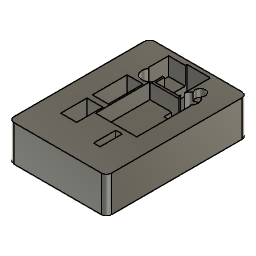
soldering jig v4 (Autodesk Fusion 360 design; units mm, degrees)
Autodesk Fusion 360 part; units mm, degrees
(part 1 of 4)
sketch "Universal_Board_Side_Mount" plane through (0, 0, 0) normal (0, 0, 1) x (1, 0, 0)
  arc A0 (2.8448, 30.9521) -> (2.7093, 31.3585) centre (2.1675, 30.9521) ccw
  arc A1 (2.2648, 29.4642) -> (2.341, 29.4642) centre (2.3029, 29.4642) ccw
  arc A2 (2.1675, 30.7715) -> (2.4836, 30.5909) centre (2.4836, 30.9577) ccw
  arc A3 (1.2192, 29.9158) -> (1.4901, 29.6448) centre (1.4902, 29.9158) ccw
  arc A4 (1.2573, 29.9158) -> (1.1811, 29.9158) centre (1.2192, 29.9158) ccw
  arc A5 (1.5804, 31.4107) -> (1.5804, 31.4869) centre (1.5804, 31.4488) ccw
  arc A6 (1.5804, 31.4488) -> (1.2192, 31.0876) centre (1.5804, 31.0876) ccw
  arc A7 (1.8637, 31.2489) -> (1.9294, 31.2875) centre (1.8965, 31.2682) ccw
  arc A8 (2.4836, 23.7652) -> (2.8448, 24.1265) centre (2.4835, 24.1265) ccw
  line L0 (2.8448, 29.6448) -> (1.4901, 29.6448)
  arc A9 (2.4836, 30.5909) -> (2.8448, 30.9521) centre (2.4836, 30.9521) ccw
  arc A10 (2.4836, 30.5528) -> (2.4836, 30.629) centre (2.4836, 30.5909) ccw
  arc A11 (2.4836, 23.8033) -> (2.4836, 23.7271) centre (2.4836, 23.7652) ccw
  arc A12 (1.2192, 31.0876) -> (1.445, 30.5457) centre (1.9824, 31.0876) ccw
  arc A13 (2.8067, 24.1265) -> (2.8829, 24.1265) centre (2.8448, 24.1265) ccw
  arc A14 (1.8965, 31.2682) -> (1.5804, 31.4488) centre (1.5804, 31.082) ccw
  arc A15 (1.4901, 29.6829) -> (1.4901, 29.6067) centre (1.4901, 29.6448) ccw
  arc A16 (2.8448, 29.6067) -> (2.8448, 29.6829) centre (2.8448, 29.6448) ccw
  arc A17 (1.4901, 29.6067) -> (1.4901, 29.6829) centre (1.4901, 29.6448) ccw
  arc A18 (1.4901, 32.7867) -> (1.4901, 32.8629) centre (1.4901, 32.8248) ccw
  line L1 (1.2192, 29.9158) -> (1.2192, 30.0061)
  arc A19 (1.2573, 30.0061) -> (1.1811, 30.0061) centre (1.2192, 30.0061) ccw
  arc A20 (1.1811, 31.0876) -> (1.2573, 31.0876) centre (1.2192, 31.0876) ccw
  arc A21 (2.8829, 24.1265) -> (2.8067, 24.1265) centre (2.8448, 24.1265) ccw
  arc A22 (2.8448, 24.1265) -> (2.7093, 24.5329) centre (2.1675, 24.1265) ccw
  arc A23 (2.7398, 24.5557) -> (2.6789, 24.51) centre (2.7093, 24.5329) ccw
  arc A24 (1.1811, 29.9158) -> (1.2573, 29.9158) centre (1.2192, 29.9158) ccw
  arc A25 (1.1811, 24.262) -> (1.2573, 24.262) centre (1.2192, 24.262) ccw
  arc A26 (2.4836, 23.7271) -> (2.4836, 23.8033) centre (2.4836, 23.7652) ccw
  arc A27 (2.4836, 30.629) -> (2.4836, 30.5528) centre (2.4836, 30.5909) ccw
  arc A28 (2.2003, 23.9652) -> (2.1346, 23.9265) centre (2.1675, 23.9459) ccw
  arc A29 (1.2192, 24.262) -> (1.445, 23.7201) centre (1.9824, 24.262) ccw
  arc A30 (2.8067, 30.9521) -> (2.8829, 30.9521) centre (2.8448, 30.9521) ccw
  arc A31 (1.4181, 23.693) -> (1.4718, 23.7471) centre (1.445, 23.7201) ccw
  arc A32 (2.032, 34.8114) -> (2.032, 34.8876) centre (2.032, 34.8495) ccw
  line L2 (2.8448, 33.4913) -> (2.7545, 33.4913)
  arc A33 (2.341, 32.5538) -> (2.2648, 32.5538) centre (2.3029, 32.5538) ccw
  arc A34 (2.3029, 34.5786) -> (2.032, 34.8495) centre (2.032, 34.5786) ccw
  arc A35 (2.8448, 33.4532) -> (2.8448, 33.5294) centre (2.8448, 33.4913) ccw
  arc A36 (1.969, 37.4483) -> (2.0047, 37.5157) centre (1.9868, 37.482) ccw
  arc A37 (1.5804, 24.6613) -> (1.5804, 24.5851) centre (1.5804, 24.6232) ccw
  arc A38 (2.134, 23.9276) -> (2.2009, 23.9641) centre (2.1674, 23.9459) ccw
  arc A39 (2.8067, 36.0444) -> (2.8829, 36.0444) centre (2.8448, 36.0444) ccw
  line L3 (2.3029, 34.127) -> (2.3029, 34.5786)
  arc A40 (2.1675, 23.9459) -> (2.4836, 23.7652) centre (2.4836, 24.1321) ccw
  arc A41 (1.2072, 39.6306) -> (1.2312, 39.5583) centre (1.2192, 39.5945) ccw
  arc A42 (2.4384, 36.4508) -> (2.1223, 36.3154) centre (2.4383, 36.0144) ccw
  line L4 (2.3029, 37.8884) -> (1.7611, 37.1659)
  arc A43 (2.341, 34.5786) -> (2.2648, 34.5786) centre (2.3029, 34.5786) ccw
  arc A44 (2.4718, 35.5839) -> (2.4953, 35.5115) centre (2.4836, 35.5477) ccw
  arc A45 (2.8829, 36.0444) -> (2.8067, 36.0444) centre (2.8448, 36.0444) ccw
  arc A46 (1.5804, 24.5851) -> (1.5804, 24.6613) centre (1.5804, 24.6232) ccw
  arc A47 (2.3029, 34.0889) -> (2.3029, 34.1651) centre (2.3029, 34.127) ccw
  arc A48 (2.8448, 41.0464) -> (2.4384, 41.4528) centre (2.4384, 41.0464) ccw
  line L5 (2.1223, 36.3154) -> (1.2192, 35.5477)
  arc A49 (1.1945, 35.5767) -> (1.2439, 35.5187) centre (1.2192, 35.5477) ccw
  arc A50 (2.4384, 36.4127) -> (2.4384, 36.4889) centre (2.4384, 36.4508) ccw
  arc A51 (2.0947, 36.3416) -> (2.1499, 36.2891) centre (2.1223, 36.3154) ccw
  arc A52 (2.7164, 33.401) -> (2.7926, 33.401) centre (2.7545, 33.401) ccw
  arc A53 (1.8637, 24.4232) -> (1.9294, 24.4619) centre (1.8966, 24.4426) ccw
  arc A54 (2.8067, 41.0464) -> (2.8829, 41.0464) centre (2.8448, 41.0464) ccw
  arc A55 (2.032, 34.8876) -> (2.032, 34.8114) centre (2.032, 34.8495) ccw
  line L6 (1.2192, 37.1659) -> (2.8448, 37.1659)
  arc A56 (2.3334, 37.8655) -> (2.2725, 37.9113) centre (2.303, 37.8884) ccw
  line L7 (2.8448, 33.401) -> (2.8448, 33.4913)
  arc A57 (2.7545, 33.4391) -> (2.7545, 33.3629) centre (2.7545, 33.401) ccw
  line L8 (2.032, 34.8495) -> (1.2192, 34.8495)
  arc A58 (2.2648, 34.127) -> (2.341, 34.127) centre (2.3029, 34.127) ccw
  arc A59 (2.4718, 40.5859) -> (2.4953, 40.5134) centre (2.4836, 40.5496) ccw
  arc A60 (1.5804, 24.6232) -> (1.2192, 24.262) centre (1.5804, 24.262) ccw
  line L9 (1.2192, 39.5944) -> (2.3029, 39.9557)
  line L10 (1.8965, 24.4426) -> (2.1675, 23.9459)
  arc A61 (2.8067, 33.401) -> (2.8829, 33.401) centre (2.8448, 33.401) ccw
  arc A62 (1.8965, 24.4426) -> (1.5804, 24.6232) centre (1.5804, 24.2564) ccw
  arc A63 (1.4901, 32.8629) -> (1.4901, 32.7867) centre (1.4901, 32.8248) ccw
  arc A64 (2.8448, 33.3629) -> (2.8448, 33.4391) centre (2.8448, 33.401) ccw
  arc A65 (2.7545, 33.5294) -> (2.7545, 33.4532) centre (2.7545, 33.4913) ccw
  arc A66 (1.93, 31.2865) -> (1.8631, 31.25) centre (1.8966, 31.2682) ccw
  arc A67 (1.2312, 39.6306) -> (1.2072, 39.5583) centre (1.2192, 39.5945) ccw
  arc A68 (1.2573, 24.262) -> (1.1811, 24.2619) centre (1.2192, 24.2619) ccw
  arc A69 (2.4384, 41.4909) -> (2.4384, 41.4147) centre (2.4384, 41.4528) ccw
  line L11 (2.3029, 39.2332) -> (1.2192, 39.5944)
  arc A70 (2.4836, 35.5477) -> (2.8448, 36.0444) centre (2.3227, 36.0444) ccw
  arc A71 (2.4836, 40.5497) -> (2.8448, 41.0464) centre (2.3227, 41.0464) ccw
  arc A72 (2.4384, 36.4889) -> (2.4384, 36.4127) centre (2.4384, 36.4508) ccw
  arc A73 (1.2192, 37.204) -> (1.2192, 37.1278) centre (1.2192, 37.1659) ccw
  arc A74 (11.3867, 7.6438) -> (11.3674, 7.6766) centre (11.3771, 7.6602) ccw
  arc A75 (1.237, 37.9221) -> (1.2014, 37.8547) centre (1.2192, 37.8884) ccw
  line L12 (11.3771, 7.6602) -> (11.6021, 7.783)
  arc A76 (2.4384, 41.4147) -> (2.4384, 41.4909) centre (2.4384, 41.4528) ccw
  arc A77 (1.7306, 37.1888) -> (1.7915, 37.1431) centre (1.761, 37.1659) ccw
  arc A78 (11.3143, 7.517) -> (11.2762, 7.517) centre (11.2953, 7.517) ccw
  arc A79 (1.2192, 34.8876) -> (1.2192, 34.8114) centre (1.2192, 34.8495) ccw
  line L13 (1.2192, 35.5477) -> (1.2192, 36.4508)
  line L14 (29.1592, 41.6532) -> (28.3803, 41.6532)
  arc A80 (11.3247, 8.0438) -> (11.3476, 8.0133) centre (11.3361, 8.0285) ccw
  arc A81 (11.3771, 7.6602) -> (11.2952, 7.517) centre (11.4614, 7.5169) ccw
  arc A82 (24.7438, 43.7776) -> (24.7438, 43.7395) centre (24.7438, 43.7585) ccw
  line L15 (25.2349, 43.7586) -> (24.7438, 43.7586)
  arc A83 (2.7926, 33.4913) -> (2.7164, 33.4913) centre (2.7545, 33.4913) ccw
  arc A84 (11.718, 7.4422) -> (11.6909, 7.469) centre (11.7044, 7.4556) ccw
  line L16 (24.9894, 43.513) -> (24.9894, 44.0041)
  line L17 (11.9084, 40.084) -> (11.9084, 40.5751)
  arc A85 (2.0947, 41.3436) -> (2.1499, 41.2911) centre (2.1223, 41.3173) ccw
  line L18 (2.1223, 41.3173) -> (1.2192, 40.5497)
  line L19 (1.2192, 40.5497) -> (1.2192, 41.4528)
  arc A86 (2.315, 39.9195) -> (2.2909, 39.9918) centre (2.303, 39.9557) ccw
  arc A87 (1.1811, 40.5497) -> (1.2573, 40.5497) centre (1.2192, 40.5497) ccw
  arc A88 (28.3803, 43.8376) -> (28.3803, 43.7868) centre (28.3803, 43.8122) ccw
  arc A89 (2.3029, 33.4081) -> (2.3029, 33.4843) centre (2.3029, 33.4462) ccw
  arc A90 (2.8448, 36.0444) -> (2.4384, 36.4508) centre (2.4384, 36.0444) ccw
  arc A91 (24.8539, 41.9615) -> (24.8539, 41.9996) centre (24.8539, 41.9806) ccw
  arc A92 (11.8893, 40.084) -> (11.9274, 40.084) centre (11.9084, 40.084) ccw
  arc A93 (25.0084, 44.0041) -> (24.9703, 44.0041) centre (24.9894, 44.0041) ccw
  line L20 (29.1592, 43.8122) -> (28.3803, 43.8122)
  arc A94 (28.3803, 41.6786) -> (28.3803, 41.6278) centre (28.3803, 41.6532) ccw
  arc A95 (2.2648, 34.5786) -> (2.341, 34.5786) centre (2.3029, 34.5786) ccw
  arc A96 (2.8829, 33.4913) -> (2.8067, 33.4913) centre (2.8448, 33.4913) ccw
  arc A97 (29.1592, 41.6278) -> (29.1592, 41.6786) centre (29.1592, 41.6532) ccw
  arc A98 (24.9703, 43.513) -> (25.0084, 43.513) centre (24.9894, 43.513) ccw
  arc A99 (1.2573, 36.4508) -> (1.1811, 36.4508) centre (1.2192, 36.4508) ccw
  arc A100 (11.5925, 7.7994) -> (11.6118, 7.7666) centre (11.6021, 7.783) ccw
  arc A101 (12.1539, 40.3105) -> (12.1539, 40.3486) centre (12.1539, 40.3295) ccw
  arc A102 (9.2329, 45.7715) -> (9.2329, 45.8096) centre (9.2329, 45.7906) ccw
  line L21 (1.2192, 37.8884) -> (1.9868, 37.482)
  arc A103 (1.1811, 35.5477) -> (1.2573, 35.5477) centre (1.2192, 35.5477) ccw
  arc A104 (11.6113, 7.7663) -> (11.593, 7.7997) centre (11.6021, 7.783) ccw
  arc A105 (24.6274, 42.2261) -> (24.5893, 42.2261) centre (24.6084, 42.2261) ccw
  arc A106 (11.6628, 40.3486) -> (11.6628, 40.3105) centre (11.6628, 40.3295) ccw
  arc A107 (1.2573, 41.4528) -> (1.1811, 41.4528) centre (1.2192, 41.4528) ccw
  arc A108 (2.8448, 37.1278) -> (2.8448, 37.204) centre (2.8448, 37.1659) ccw
  line L22 (1.2192, 34.127) -> (2.3029, 34.127)
  arc A109 (29.1592, 43.7868) -> (29.1592, 43.8376) centre (29.1592, 43.8122) ccw
  arc A110 (2.8829, 41.0464) -> (2.8067, 41.0464) centre (2.8448, 41.0464) ccw
  line L23 (2.7545, 33.401) -> (2.8448, 33.401)
  arc A111 (25.2349, 43.7395) -> (25.2349, 43.7776) centre (25.2349, 43.7585) ccw
  line L24 (2.7545, 33.4913) -> (2.7545, 33.401)
  arc A112 (24.3628, 41.9996) -> (24.3628, 41.9615) centre (24.3628, 41.9806) ccw
  line L25 (7.9629, 42.3616) -> (7.4718, 42.3616)
  arc A113 (7.4718, 42.3806) -> (7.4718, 42.3425) centre (7.4718, 42.3616) ccw
  arc A114 (2.2909, 39.197) -> (2.315, 39.2693) centre (2.303, 39.2332) ccw
  arc A115 (11.3679, 7.6769) -> (11.3862, 7.6435) centre (11.3771, 7.6602) ccw
  arc A116 (1.2192, 34.1651) -> (1.2192, 34.0889) centre (1.2192, 34.127) ccw
  arc A117 (2.147, 36.2863) -> (2.0976, 36.3444) centre (2.1223, 36.3154) ccw
  arc A118 (11.2762, 7.517) -> (11.3143, 7.517) centre (11.2953, 7.517) ccw
  line L26 (24.6084, 41.735) -> (24.6084, 42.2261)
  arc A119 (1.2192, 33.4843) -> (1.2192, 33.4081) centre (1.2192, 33.4462) ccw
  line L27 (9.2329, 45.7906) -> (8.7418, 45.7906)
  line L28 (9.8677, 8.0899) -> (9.8268, 8.0899)
  arc A120 (10.3484, 7.8444) -> (10.3103, 7.8444) centre (10.3294, 7.8444) ccw
  arc A121 (7.9629, 42.3425) -> (7.9629, 42.3806) centre (7.9629, 42.3616) ccw
  arc A122 (11.6649, 7.9262) -> (11.703, 7.9262) centre (11.6839, 7.9262) ccw
  arc A123 (8.8056, 7.6807) -> (8.8437, 7.6807) centre (8.8247, 7.6807) ccw
  line L29 (7.9629, 15.9456) -> (7.4718, 15.9456)
  arc A124 (11.5203, 8.0709) -> (11.5203, 8.1089) centre (11.5203, 8.0899) ccw
  arc A125 (11.4589, 7.3723) -> (11.4589, 7.3343) centre (11.4589, 7.3533) ccw
  arc A126 (9.4328, 7.3723) -> (9.4328, 7.3342) centre (9.4328, 7.3533) ccw
  arc A127 (9.5774, 7.4761) -> (9.6155, 7.4761) centre (9.5965, 7.4761) ccw
  arc A128 (9.152, 7.6807) -> (8.8246, 7.6807) centre (8.9883, 7.6807) ccw
  arc A129 (11.6021, 7.783) -> (11.684, 7.9262) centre (11.5178, 7.9263) ccw
  arc A130 (1.1945, 40.5787) -> (1.2439, 40.5207) centre (1.2192, 40.5497) ccw
  arc A131 (10.7761, 7.8253) -> (10.7762, 7.8634) centre (10.7761, 7.8444) ccw
  line L30 (8.8246, 7.6807) -> (8.8246, 7.5988)
  arc A132 (11.684, 7.9262) -> (11.5203, 8.0899) centre (11.5203, 7.9262) ccw
  arc A133 (11.2952, 7.517) -> (11.4589, 7.3533) centre (11.4589, 7.517) ccw
  line L31 (24.8539, 41.9806) -> (24.3628, 41.9806)
  line L32 (10.3294, 7.3533) -> (10.3294, 7.8444)
  arc A134 (9.171, 7.6807) -> (9.1329, 7.6807) centre (9.1519, 7.6807) ccw
  line L33 (12.1539, 40.3296) -> (11.6628, 40.3296)
  arc A135 (10.3103, 7.3533) -> (10.3484, 7.3533) centre (10.3294, 7.3533) ccw
  arc A136 (9.9714, 7.3533) -> (10.0095, 7.3533) centre (9.9904, 7.3533) ccw
  arc A137 (10.6724, 7.7216) -> (10.6343, 7.7216) centre (10.6534, 7.7216) ccw
  line L34 (9.9904, 7.3533) -> (9.9904, 7.9671)
  line L35 (10.6534, 7.7216) -> (10.6534, 7.3533)
  arc A138 (8.7418, 45.8096) -> (8.7418, 45.7715) centre (8.7418, 45.7906) ccw
  arc A139 (7.4718, 15.9646) -> (7.4718, 15.9265) centre (7.4718, 15.9455) ccw
  arc A140 (9.4328, 7.8634) -> (9.4328, 7.8253) centre (9.4328, 7.8444) ccw
  arc A141 (7.9629, 15.9265) -> (7.9629, 15.9646) centre (7.9629, 15.9455) ccw
  arc A142 (9.8677, 8.109) -> (9.8677, 8.0709) centre (9.8677, 8.0899) ccw
  arc A143 (11.4589, 7.3343) -> (11.4589, 7.3723) centre (11.4589, 7.3533) ccw
  arc A144 (11.703, 7.9262) -> (11.6649, 7.9262) centre (11.6839, 7.9262) ccw
  arc A145 (9.0292, 7.3723) -> (9.0292, 7.3342) centre (9.0292, 7.3533) ccw
  arc A146 (10.6343, 7.7216) -> (10.6724, 7.7216) centre (10.6534, 7.7216) ccw
  arc A147 (10.3499, 8.0299) -> (10.3499, 8.068) centre (10.3499, 8.0489) ccw
  arc A148 (10.2899, 8.049) -> (10.328, 8.049) centre (10.309, 8.049) ccw
  arc A149 (8.8246, 7.3723) -> (8.8246, 7.3342) centre (8.8246, 7.3533) ccw
  arc A150 (10.6343, 7.3533) -> (10.6724, 7.3533) centre (10.6534, 7.3533) ccw
  arc A151 (10.3089, 8.109) -> (10.3089, 8.0709) centre (10.3089, 8.0899) ccw
  line L36 (9.5965, 8.0899) -> (9.5965, 7.4761)
  arc A152 (10.9617, 7.3533) -> (10.9998, 7.3533) centre (10.9808, 7.3533) ccw
  arc A153 (10.3499, 8.0709) -> (10.3499, 8.109) centre (10.3499, 8.0899) ccw
  line L37 (10.0723, 7.8444) -> (9.8268, 7.8444)
  line L38 (10.9808, 7.8444) -> (10.7762, 7.8444)
  line L39 (10.3089, 8.0899) -> (10.3089, 8.049)
  arc A154 (9.9714, 7.9671) -> (10.0095, 7.9671) centre (9.9904, 7.9671) ccw
  arc A155 (2.147, 41.2883) -> (2.0976, 41.3464) centre (2.1223, 41.3173) ccw
  arc A156 (11.5203, 8.0899) -> (11.3361, 8.0285) centre (11.5203, 7.7829) ccw
  arc A157 (2.4384, 41.4528) -> (2.1223, 41.3173) centre (2.4384, 41.0163) ccw
  arc A158 (11.5203, 8.109) -> (11.5203, 8.0709) centre (11.5203, 8.0899) ccw
  arc A159 (10.0095, 7.9671) -> (9.9714, 7.9671) centre (9.9904, 7.9671) ccw
  arc A160 (9.6155, 8.0899) -> (9.5774, 8.0899) centre (9.5965, 8.0899) ccw
  arc A161 (11.9274, 40.5751) -> (11.8893, 40.5751) centre (11.9084, 40.5751) ccw
  arc A162 (9.171, 7.4761) -> (9.1329, 7.4761) centre (9.1519, 7.4761) ccw
  line L40 (10.3499, 8.049) -> (10.3499, 8.0899)
  arc A163 (9.1329, 7.4761) -> (9.171, 7.4761) centre (9.1519, 7.4761) ccw
  arc A164 (9.1329, 7.6807) -> (9.171, 7.6807) centre (9.1519, 7.6807) ccw
  arc A165 (24.5893, 41.735) -> (24.6274, 41.735) centre (24.6084, 41.735) ccw
  arc A166 (11.4589, 7.3533) -> (11.7044, 7.4556) centre (11.4589, 7.6991) ccw
  arc A167 (9.6155, 7.4761) -> (9.5774, 7.4761) centre (9.5965, 7.4761) ccw
  line L41 (9.6783, 7.8444) -> (9.4328, 7.8444)
  line L42 (9.4737, 7.3533) -> (9.4328, 7.3533)
  arc A168 (10.9998, 8.0899) -> (10.9617, 8.0899) centre (10.9808, 8.0899) ccw
  arc A169 (10.328, 8.0899) -> (10.2899, 8.0899) centre (10.309, 8.0899) ccw
  arc A170 (7.2818, 28.0698) -> (7.2513, 28.047) centre (7.2666, 28.0584) ccw
  arc A171 (9.4737, 7.3723) -> (9.4737, 7.3342) centre (9.4737, 7.3533) ccw
  arc A172 (9.8268, 7.8634) -> (9.8268, 7.8253) centre (9.8268, 7.8444) ccw
  arc A173 (7.1642, 27.7296) -> (7.1642, 27.6915) centre (7.1642, 27.7106) ccw
  arc A174 (9.5765, 9.5032) -> (9.6146, 9.5032) centre (9.5956, 9.5032) ccw
  arc A175 (6.6103, 27.9356) -> (6.5723, 27.9356) centre (6.5913, 27.9356) ccw
  arc A176 (7.0374, 27.8021) -> (7.0046, 27.7827) centre (7.021, 27.7924) ccw
  arc A177 (7.0043, 27.7833) -> (7.0377, 27.8015) centre (7.021, 27.7924) ccw
  arc A178 (7.3469, 27.8742) -> (7.3088, 27.8742) centre (7.3278, 27.8742) ccw
  arc A179 (8.2625, 7.8444) -> (8.2244, 7.8444) centre (8.2434, 7.8444) ccw
  line L43 (10.3089, 8.049) -> (10.3499, 8.049)
  arc A180 (9.6131, 10.8306) -> (9.578, 10.8159) centre (9.5956, 10.8233) ccw
  arc A181 (7.7329, 7.5756) -> (7.747, 7.5402) centre (7.7399, 7.5579) ccw
  arc A182 (7.021, 27.7924) -> (7.1642, 27.7106) centre (7.1642, 27.8768) ccw
  arc A183 (10.7762, 7.8634) -> (10.7762, 7.8253) centre (10.7762, 7.8444) ccw
  arc A184 (7.7806, 7.3723) -> (7.7811, 7.3343) centre (7.7809, 7.3533) ccw
  line L44 (10.9808, 7.3533) -> (10.9808, 8.0899)
  arc A185 (7.1642, 27.7106) -> (7.3279, 27.8742) centre (7.1642, 27.8743) ccw
  arc A186 (6.9149, 28.0266) -> (6.8815, 28.0083) centre (6.8982, 28.0175) ccw
  arc A187 (9.6783, 7.8253) -> (9.6783, 7.8634) centre (9.6783, 7.8444) ccw
  line L45 (7.0824, 28.3264) -> (7.0824, 28.5719)
  line L46 (9.8002, 10.3322) -> (9.5956, 10.8233)
  arc A188 (9.152, 7.5798) -> (9.152, 7.6179) centre (9.152, 7.5989) ccw
  arc A189 (8.8437, 7.6807) -> (8.8056, 7.6807) centre (8.8247, 7.6807) ccw
  arc A190 (10.3308, 8.049) -> (10.3689, 8.049) centre (10.3498, 8.049) ccw
  arc A191 (6.755, 28.1184) -> (6.755, 28.0803) centre (6.755, 28.0994) ccw
  arc A192 (10.3089, 8.068) -> (10.3089, 8.0299) centre (10.3089, 8.0489) ccw
  line L47 (9.152, 7.4761) -> (9.152, 7.6807)
  arc A193 (10.9808, 7.8253) -> (10.9808, 7.8634) centre (10.9808, 7.8444) ccw
  arc A194 (9.4737, 7.3533) -> (9.5965, 7.4761) centre (9.4737, 7.4761) ccw
  arc A195 (7.9375, 7.6574) -> (7.9516, 7.6221) centre (7.9446, 7.6397) ccw
  arc A196 (10.3689, 8.0899) -> (10.3308, 8.0899) centre (10.3498, 8.0899) ccw
  arc A197 (9.5765, 8.6741) -> (9.6146, 8.6741) centre (9.5956, 8.6741) ccw
  arc A198 (7.7117, 7.8208) -> (7.7273, 7.7861) centre (7.7195, 7.8035) ccw
  arc A199 (7.747, 7.5402) -> (7.7329, 7.5756) centre (7.74, 7.5579) ccw
  arc A200 (9.0292, 7.3533) -> (9.152, 7.4761) centre (9.0292, 7.4761) ccw
  arc A201 (9.6131, 10.8159) -> (9.578, 10.8306) centre (9.5955, 10.8232) ccw
  arc A202 (6.8982, 28.0175) -> (6.755, 28.0993) centre (6.755, 27.9331) ccw
  arc A203 (9.9904, 7.9671) -> (9.8677, 8.0899) centre (9.8676, 7.9671) ccw
  line L48 (10.3499, 8.0899) -> (10.3089, 8.0899)
  arc A204 (9.8268, 8.109) -> (9.8268, 8.0709) centre (9.8268, 8.0899) ccw
  arc A205 (10.0723, 7.8253) -> (10.0723, 7.8634) centre (10.0723, 7.8444) ccw
  arc A206 (10.7762, 7.8444) -> (10.6534, 7.7216) centre (10.7762, 7.7216) ccw
  arc A207 (7.3089, 27.8742) -> (7.3469, 27.8742) centre (7.3279, 27.8742) ccw
  line L49 (7.7399, 7.5579) -> (7.9446, 7.6398)
  arc A208 (7.9446, 7.6398) -> (7.9036, 7.8444) centre (7.9052, 7.7383) ccw
  line L50 (8.8246, 7.3533) -> (9.0292, 7.3533)
  arc A209 (9.4737, 7.3342) -> (9.4737, 7.3723) centre (9.4737, 7.3533) ccw
  arc A210 (6.8818, 28.0078) -> (6.9146, 28.0271) centre (6.8982, 28.0175) ccw
  arc A211 (7.3279, 27.8742) -> (7.2665, 28.0584) centre (7.0209, 27.8742) ccw
  arc A212 (9.8677, 8.0709) -> (9.8677, 8.109) centre (9.8677, 8.0899) ccw
  line L51 (9.5956, 8.6741) -> (9.5956, 9.1652)
  arc A213 (9.0292, 7.3342) -> (9.0292, 7.3723) centre (9.0292, 7.3533) ccw
  arc A214 (7.1642, 27.6915) -> (7.1642, 27.7296) centre (7.1642, 27.7106) ccw
  line L52 (6.8982, 28.0175) -> (7.021, 27.7924)
  arc A215 (7.1014, 28.5719) -> (7.0633, 28.5719) centre (7.0824, 28.5719) ccw
  arc A216 (7.9516, 7.6221) -> (7.9375, 7.6574) centre (7.9445, 7.6398) ccw
  arc A217 (6.9187, 28.8527) -> (6.9187, 29.1801) centre (6.9187, 29.0164) ccw
  arc A218 (6.7141, 28.4272) -> (6.7141, 28.3891) centre (6.7141, 28.4081) ccw
  arc A219 (6.5913, 28.531) -> (6.7141, 28.4082) centre (6.7141, 28.531) ccw
  line L53 (6.3458, 30.1735) -> (7.0824, 30.1735)
  arc A220 (6.6104, 30.3781) -> (6.5723, 30.3781) centre (6.5914, 30.3781) ccw
  arc A221 (7.7399, 7.5579) -> (7.7809, 7.3533) centre (7.7793, 7.4594) ccw
  line L54 (9.5956, 10.8233) -> (9.3909, 10.3322)
  arc A222 (6.755, 28.0803) -> (6.755, 28.1184) centre (6.755, 28.0994) ccw
  arc A223 (8.489, 7.8253) -> (8.489, 7.8634) centre (8.489, 7.8444) ccw
  line L55 (9.5956, 9.5032) -> (9.5956, 9.9942)
  arc A224 (6.7141, 28.8336) -> (6.7141, 28.8717) centre (6.7141, 28.8527) ccw
  arc A225 (7.0824, 30.3781) -> (6.9596, 30.5009) centre (6.9596, 30.3781) ccw
  arc A226 (6.5913, 28.9754) -> (6.7141, 28.8527) centre (6.7141, 28.9755) ccw
  arc A227 (6.7141, 29.8235) -> (6.7141, 29.8616) centre (6.7141, 29.8426) ccw
  arc A228 (6.9187, 29.161) -> (6.9187, 29.1991) centre (6.9187, 29.1801) ccw
  line L56 (6.8368, 29.1801) -> (6.8368, 28.8527)
  arc A229 (9.6146, 9.9942) -> (9.5765, 9.9942) centre (9.5956, 9.9942) ccw
  arc A230 (7.0633, 30.3781) -> (7.1014, 30.3781) centre (7.0824, 30.3781) ccw
  arc A231 (7.0824, 29.7197) -> (6.9596, 29.8425) centre (6.9596, 29.7197) ccw
  line L57 (6.9596, 29.8425) -> (6.7141, 29.8425)
  arc A232 (7.7809, 7.3533) -> (8.0059, 7.3942) centre (7.7711, 8.0468) ccw
  arc A233 (6.6802, 27.6766) -> (6.707, 27.7036) centre (6.6936, 27.6901) ccw
  arc A234 (7.9034, 7.8634) -> (7.9039, 7.8253) centre (7.9036, 7.8444) ccw
  arc A235 (6.7141, 30.5009) -> (6.5913, 30.3781) centre (6.7141, 30.3781) ccw
  line L58 (6.5913, 29.1801) -> (6.5913, 28.9754)
  arc A236 (9.7826, 10.3249) -> (9.8178, 10.3395) centre (9.8002, 10.3322) ccw
  arc A237 (7.9039, 7.8253) -> (7.9034, 7.8634) centre (7.9036, 7.8444) ccw
  line L59 (8.2435, 7.8444) -> (8.2435, 7.7625)
  arc A238 (8.2244, 7.7625) -> (8.2625, 7.7625) centre (8.2434, 7.7625) ccw
  arc A239 (6.5723, 28.9754) -> (6.6104, 28.9754) centre (6.5914, 28.9754) ccw
  arc A240 (6.8559, 29.1801) -> (6.8178, 29.1801) centre (6.8369, 29.1801) ccw
  arc A241 (8.5081, 7.8444) -> (8.47, 7.8444) centre (8.4891, 7.8444) ccw
  arc A242 (6.5723, 30.1735) -> (6.6104, 30.1735) centre (6.5914, 30.1735) ccw
  arc A243 (6.5723, 28.531) -> (6.6104, 28.531) centre (6.5914, 28.531) ccw
  arc A244 (8.8056, 7.5988) -> (8.8437, 7.5988) centre (8.8247, 7.5988) ccw
  line L60 (8.489, 7.8444) -> (8.2435, 7.8444)
  arc A245 (8.2435, 7.8634) -> (8.2435, 7.8253) centre (8.2435, 7.8444) ccw
  arc A246 (8.8246, 7.6179) -> (8.8246, 7.5798) centre (8.8246, 7.5989) ccw
  arc A247 (9.6146, 9.1652) -> (9.5765, 9.1652) centre (9.5956, 9.1652) ccw
  line L61 (6.5913, 30.3781) -> (6.5913, 30.1735)
  arc A248 (6.5723, 29.5151) -> (6.6104, 29.5151) centre (6.5914, 29.5151) ccw
  arc A249 (9.3734, 10.3395) -> (9.4085, 10.3249) centre (9.391, 10.3322) ccw
  line L62 (8.489, 7.3533) -> (8.489, 7.8444)
  arc A250 (6.5722, 29.7197) -> (6.6103, 29.7197) centre (6.5913, 29.7197) ccw
  line L63 (7.0824, 29.5151) -> (7.0824, 29.7197)
  arc A251 (6.3458, 30.1926) -> (6.3458, 30.1545) centre (6.3458, 30.1735) ccw
  arc A252 (7.0633, 28.3264) -> (7.1014, 28.3264) centre (7.0824, 28.3264) ccw
  arc A253 (7.1014, 30.3781) -> (7.0633, 30.3781) centre (7.0824, 30.3781) ccw
  line L64 (6.3458, 29.5151) -> (7.0824, 29.5151)
  arc A254 (6.755, 28.0993) -> (6.5913, 27.9356) centre (6.755, 27.9356) ccw
  arc A255 (7.9036, 7.8444) -> (7.7195, 7.8034) centre (7.9105, 7.3796) ccw
  arc A256 (6.5913, 27.9356) -> (6.6936, 27.6901) centre (6.9371, 27.9356) ccw
  arc A257 (7.7811, 7.3343) -> (7.7806, 7.3723) centre (7.7809, 7.3533) ccw
  arc A258 (6.7141, 30.5199) -> (6.7141, 30.4818) centre (6.7141, 30.5008) ccw
  arc A259 (7.0824, 29.4961) -> (7.0824, 29.5342) centre (7.0824, 29.5152) ccw
  arc A260 (8.0124, 7.3763) -> (7.9995, 7.4121) centre (8.0059, 7.3942) ccw
  arc A261 (8.47, 7.3533) -> (8.5081, 7.3533) centre (8.4891, 7.3533) ccw
  arc A262 (6.6104, 28.5719) -> (6.5723, 28.5719) centre (6.5914, 28.5719) ccw
  arc A263 (6.6104, 29.7197) -> (6.5723, 29.7197) centre (6.5914, 29.7197) ccw
  arc A264 (6.3458, 29.5342) -> (6.3458, 29.4961) centre (6.3458, 29.5152) ccw
  arc A265 (6.5722, 27.9356) -> (6.6103, 27.9356) centre (6.5913, 27.9356) ccw
  line L65 (8.8246, 7.5988) -> (9.152, 7.5988)
  line L66 (7.0824, 30.1735) -> (7.0824, 30.3781)
  arc A266 (6.9596, 30.5199) -> (6.9596, 30.4818) centre (6.9596, 30.5008) ccw
  arc A267 (6.7141, 30.8224) -> (6.7141, 30.7843) centre (6.7141, 30.8034) ccw
  arc A268 (7.6006, 47.046) -> (7.614, 47.0103) centre (7.6073, 47.0282) ccw
  arc A269 (7.9414, 47.1331) -> (7.928, 47.1688) centre (7.9347, 47.151) ccw
  arc A270 (6.5913, 30.9262) -> (6.7141, 30.8034) centre (6.7141, 30.9262) ccw
  arc A271 (8.103, 47.378) -> (8.0937, 47.415) centre (8.0983, 47.3965) ccw
  arc A272 (6.6104, 29.1801) -> (6.5723, 29.1801) centre (6.5914, 29.1801) ccw
  arc A273 (6.7141, 28.3891) -> (6.7141, 28.4272) centre (6.7141, 28.4081) ccw
  arc A274 (6.8178, 28.8527) -> (6.8559, 28.8527) centre (6.8369, 28.8527) ccw
  arc A275 (6.9596, 30.4818) -> (6.9596, 30.5199) centre (6.9596, 30.5008) ccw
  arc A276 (6.6104, 28.9754) -> (6.5723, 28.9754) centre (6.5914, 28.9754) ccw
  arc A277 (6.7141, 30.7843) -> (6.7141, 30.8224) centre (6.7141, 30.8034) ccw
  arc A278 (6.5723, 30.9262) -> (6.6104, 30.9262) centre (6.5914, 30.9262) ccw
  line L67 (8.0984, 46.9054) -> (7.6073, 47.0282)
  arc A279 (6.6104, 30.9262) -> (6.5723, 30.9262) centre (6.5914, 30.9262) ccw
  arc A280 (7.928, 47.1331) -> (7.9414, 47.1688) centre (7.9347, 47.1509) ccw
  arc A281 (8.3248, 45.7972) -> (8.3629, 45.7972) centre (8.3438, 45.7972) ccw
  arc A282 (6.9187, 31.1498) -> (6.9187, 31.1117) centre (6.9187, 31.1307) ccw
  line L68 (8.3439, 45.5926) -> (8.3439, 45.7972)
  arc A283 (7.771, 46.2992) -> (7.771, 46.2611) centre (7.771, 46.2801) ccw
  arc A284 (6.5722, 30.3781) -> (6.6103, 30.3781) centre (6.5913, 30.3781) ccw
  line L69 (7.3279, 28.4082) -> (6.7141, 28.4082)
  arc A285 (7.1014, 29.7197) -> (7.0633, 29.7197) centre (7.0824, 29.7197) ccw
  arc A286 (6.6104, 28.531) -> (6.5723, 28.531) centre (6.5914, 28.531) ccw
  arc A287 (8.3439, 45.5736) -> (8.3439, 45.6117) centre (8.3439, 45.5926) ccw
  arc A288 (7.9347, 46.5885) -> (7.9347, 46.6266) centre (7.9347, 46.6076) ccw
  arc A289 (6.7141, 30.4818) -> (6.7141, 30.5199) centre (6.7141, 30.5008) ccw
  arc A290 (7.0824, 30.1545) -> (7.0824, 30.1926) centre (7.0824, 30.1735) ccw
  line L70 (6.9187, 29.1801) -> (6.8368, 29.1801)
  arc A291 (7.0633, 31.4664) -> (7.1014, 31.4664) centre (7.0824, 31.4664) ccw
  arc A292 (6.8559, 31.1308) -> (6.8178, 31.1308) centre (6.8369, 31.1308) ccw
  arc A293 (6.9187, 31.1117) -> (6.9187, 31.1498) centre (6.9187, 31.1307) ccw
  arc A294 (7.3279, 28.3891) -> (7.3279, 28.4272) centre (7.3279, 28.4081) ccw
  arc A295 (7.0824, 31.6928) -> (7.0824, 31.7309) centre (7.0824, 31.7118) ccw
  line L71 (7.6073, 45.5926) -> (8.3439, 45.5926)
  arc A296 (6.7141, 28.8717) -> (6.7141, 28.8336) centre (6.7141, 28.8527) ccw
  arc A297 (6.9187, 28.8717) -> (6.9187, 28.8336) centre (6.9187, 28.8527) ccw
  arc A298 (7.0633, 29.5151) -> (7.1014, 29.5151) centre (7.0824, 29.5151) ccw
  line L72 (6.9596, 30.5009) -> (6.7141, 30.5009)
  line L73 (6.7141, 28.8527) -> (6.9187, 28.8527)
  arc A299 (6.7141, 29.8425) -> (6.5913, 29.7197) centre (6.7141, 29.7197) ccw
  line L74 (7.9347, 47.1509) -> (7.6073, 47.2737)
  line L75 (6.5913, 28.531) -> (6.5913, 28.5719)
  arc A300 (6.8368, 29.1991) -> (6.8368, 29.161) centre (6.8368, 29.1801) ccw
  arc A301 (7.9156, 45.7972) -> (7.9537, 45.7972) centre (7.9347, 45.7972) ccw
  line L76 (6.8368, 31.1308) -> (6.8368, 30.8034)
  arc A302 (7.6119, 47.0467) -> (7.6027, 47.0097) centre (7.6073, 47.0282) ccw
  arc A303 (6.9187, 30.8034) -> (6.9187, 31.1308) centre (6.9187, 30.9671) ccw
  arc A304 (7.9347, 46.6266) -> (7.9347, 46.5885) centre (7.9347, 46.6076) ccw
  line L77 (7.6073, 47.0282) -> (7.9347, 47.1509)
  arc A305 (6.9187, 28.8336) -> (6.9187, 28.8717) centre (6.9187, 28.8527) ccw
  arc A306 (6.9187, 29.1991) -> (6.9187, 29.161) centre (6.9187, 29.1801) ccw
  arc A307 (7.0633, 30.1735) -> (7.1014, 30.1735) centre (7.0824, 30.1735) ccw
  line L78 (6.7141, 30.8034) -> (6.9187, 30.8034)
  arc A308 (7.614, 47.2915) -> (7.6006, 47.2559) centre (7.6073, 47.2737) ccw
  line L79 (7.6073, 47.2737) -> (8.0984, 47.3965)
  arc A309 (6.7141, 29.8616) -> (6.7141, 29.8235) centre (6.7141, 29.8426) ccw
  arc A310 (7.0633, 29.7197) -> (7.1014, 29.7197) centre (7.0824, 29.7197) ccw
  arc A311 (7.771, 46.2611) -> (7.771, 46.2992) centre (7.771, 46.2801) ccw
  arc A312 (6.8178, 30.8034) -> (6.8559, 30.8034) centre (6.8369, 30.8034) ccw
  line L80 (7.0824, 31.4664) -> (7.0824, 31.7119)
  arc A313 (6.9596, 29.8235) -> (6.9596, 29.8616) centre (6.9596, 29.8426) ccw
  line L81 (6.5913, 29.7197) -> (6.5913, 29.5151)
  arc A314 (6.9596, 29.8616) -> (6.9596, 29.8235) centre (6.9596, 29.8426) ccw
  line L82 (7.771, 46.2801) -> (7.9347, 46.2801)
  line L83 (8.0984, 48.6029) -> (8.0165, 48.6029)
  arc A315 (11.49, 50.0761) -> (11.5281, 50.0761) centre (11.5091, 50.0761) ccw
  arc A316 (8.3439, 45.7972) -> (7.9347, 45.7972) centre (8.1393, 45.7972) ccw
  line L84 (7.7301, 47.6944) -> (7.9347, 47.6944)
  arc A317 (10.964, 50.6431) -> (11.0003, 50.6549) centre (10.9822, 50.649) ccw
  line L85 (7.9347, 48.0218) -> (7.8528, 48.0218)
  line L86 (7.9347, 45.7972) -> (7.9347, 45.5926)
  arc A318 (10.6488, 50.4977) -> (10.6198, 50.473) centre (10.6343, 50.4854) ccw
  line L87 (7.8528, 48.0218) -> (7.8528, 47.6944)
  line L88 (11.7137, 50.649) -> (11.5091, 50.8127)
  arc A319 (11.7018, 50.6341) -> (11.7256, 50.6639) centre (11.7137, 50.649) ccw
  arc A320 (10.6212, 50.4715) -> (10.6475, 50.4991) centre (10.6344, 50.4853) ccw
  arc A321 (8.3248, 45.5926) -> (8.3629, 45.5926) centre (8.3438, 45.5926) ccw
  arc A322 (6.9187, 30.7843) -> (6.9187, 30.8224) centre (6.9187, 30.8034) ccw
  arc A323 (7.6264, 47.8172) -> (7.5883, 47.8172) centre (7.6074, 47.8172) ccw
  line L89 (6.5913, 31.4664) -> (7.0824, 31.4664)
  arc A324 (10.5539, 50.6286) -> (10.592, 50.6286) centre (10.573, 50.6286) ccw
  arc A325 (7.771, 46.5885) -> (7.771, 46.6266) centre (7.771, 46.6076) ccw
  arc A326 (11.5281, 50.8127) -> (11.49, 50.8127) centre (11.5091, 50.8127) ccw
  arc A327 (10.9822, 50.0571) -> (10.9822, 50.0952) centre (10.9822, 50.0762) ccw
  arc A328 (9.9736, 50.5732) -> (9.9374, 50.5611) centre (9.9555, 50.5671) ccw
  arc A329 (8.0984, 48.5839) -> (8.0984, 48.622) centre (8.0984, 48.603) ccw
  line L90 (7.0824, 31.7119) -> (7.0005, 31.7119)
  arc A330 (8.0793, 48.3574) -> (8.1174, 48.3574) centre (8.0983, 48.3574) ccw
  line L91 (8.0984, 48.3574) -> (8.0984, 48.6029)
  arc A331 (7.771, 46.6075) -> (7.771, 46.2801) centre (7.771, 46.4438) ccw
  arc A332 (10.1011, 50.0701) -> (10.1373, 50.0821) centre (10.1192, 50.0761) ccw
  arc A333 (7.6073, 45.6117) -> (7.6073, 45.5736) centre (7.6073, 45.5926) ccw
  arc A334 (7.8528, 48.0408) -> (7.8528, 48.0027) centre (7.8528, 48.0217) ccw
  line L92 (12.2894, 50.117) -> (12.2894, 50.6081)
  line L93 (11.7137, 50.0761) -> (11.3045, 50.0761)
  line L94 (11.0109, 43.6316) -> (10.5198, 43.6316)
  line L95 (6.5913, 31.1308) -> (6.5913, 30.9262)
  arc A335 (8.0984, 48.3383) -> (8.0984, 48.3764) centre (8.0984, 48.3573) ccw
  line L96 (10.2829, 50.5672) -> (10.1192, 50.0761)
  line L97 (10.1192, 50.0761) -> (9.9555, 50.5672)
  arc A336 (7.1014, 31.7119) -> (7.0633, 31.7119) centre (7.0824, 31.7119) ccw
  arc A337 (7.6027, 47.2922) -> (7.6119, 47.2552) centre (7.6073, 47.2737) ccw
  line L98 (7.9347, 46.6075) -> (7.771, 46.6075)
  arc A338 (10.9822, 50.649) -> (10.7571, 50.8127) centre (10.7571, 50.5761) ccw
  arc A339 (7.9537, 45.7972) -> (7.9156, 45.7972) centre (7.9347, 45.7972) ccw
  arc A340 (10.7571, 50.8317) -> (10.7571, 50.7937) centre (10.7571, 50.8127) ccw
  arc A341 (10.5198, 43.6506) -> (10.5198, 43.6125) centre (10.5198, 43.6315) ccw
  arc A342 (7.0005, 31.7309) -> (7.0005, 31.6928) centre (7.0005, 31.7118) ccw
  arc A343 (7.6264, 48.0218) -> (7.5883, 48.0218) centre (7.6074, 48.0218) ccw
  arc A344 (8.0937, 46.8869) -> (8.103, 46.9239) centre (8.0984, 46.9054) ccw
  arc A345 (11.521, 50.8276) -> (11.4972, 50.7978) centre (11.5091, 50.8127) ccw
  arc A346 (12.0438, 50.3816) -> (12.0438, 50.3435) centre (12.0438, 50.3626) ccw
  arc A347 (6.6104, 31.1308) -> (6.5723, 31.1308) centre (6.5914, 31.1308) ccw
  line L99 (11.5091, 50.8127) -> (11.5091, 50.0761)
  arc A348 (10.7571, 50.8127) -> (10.5729, 50.6286) centre (10.7571, 50.6285) ccw
  arc A349 (7.9347, 46.2611) -> (7.9347, 46.2992) centre (7.9347, 46.2801) ccw
  arc A350 (6.8368, 31.1498) -> (6.8368, 31.1117) centre (6.8368, 31.1307) ccw
  arc A351 (8.3629, 45.7972) -> (8.3248, 45.7972) centre (8.3438, 45.7972) ccw
  arc A352 (10.1011, 50.0821) -> (10.1373, 50.0701) centre (10.1192, 50.0761) ccw
  arc A353 (6.9187, 30.8224) -> (6.9187, 30.7843) centre (6.9187, 30.8034) ccw
  arc A354 (7.771, 46.6266) -> (7.771, 46.5885) centre (7.771, 46.6076) ccw
  arc A355 (7.9347, 46.2801) -> (7.9347, 46.6075) centre (7.9347, 46.4438) ccw
  arc A356 (7.9156, 45.5926) -> (7.9537, 45.5926) centre (7.9347, 45.5926) ccw
  arc A357 (6.5913, 31.4854) -> (6.5913, 31.4473) centre (6.5913, 31.4664) ccw
  arc A358 (7.0824, 31.4473) -> (7.0824, 31.4854) centre (7.0824, 31.4664) ccw
  line L100 (7.6073, 48.0218) -> (7.6073, 47.8172)
  line L101 (6.9187, 31.1308) -> (6.8368, 31.1308)
  arc A359 (7.9347, 46.2992) -> (7.9347, 46.2611) centre (7.9347, 46.2801) ccw
  arc A360 (10.5729, 50.6286) -> (10.6343, 50.4853) centre (10.7707, 50.6286) ccw
  line L102 (16.4719, 15.6958) -> (16.4719, 16.105)
  arc A361 (7.9347, 47.6753) -> (7.9347, 47.7134) centre (7.9347, 47.6944) ccw
  arc A362 (14.9113, 15.5131) -> (14.9113, 15.5512) centre (14.9113, 15.5321) ccw
  arc A363 (7.5883, 47.8172) -> (7.6264, 47.8172) centre (7.6074, 47.8172) ccw
  arc A364 (12.5349, 50.3435) -> (12.5349, 50.3816) centre (12.5349, 50.3626) ccw
  arc A365 (7.7301, 47.7134) -> (7.7301, 47.6753) centre (7.7301, 47.6944) ccw
  arc A366 (10.9677, 50.0638) -> (10.9967, 50.0884) centre (10.9822, 50.0761) ccw
  arc A367 (14.4831, 16.0641) -> (14.5212, 16.0641) centre (14.5022, 16.0641) ccw
  arc A368 (11.9024, 15.8361) -> (11.9171, 15.801) centre (11.9097, 15.8186) ccw
  arc A369 (16.4529, 15.6958) -> (16.491, 15.6958) centre (16.4719, 15.6958) ccw
  arc A370 (16.3082, 16.2877) -> (16.3082, 16.2496) centre (16.3082, 16.2687) ccw
  line L103 (15.2824, 15.5321) -> (15.2824, 16.2687)
  line L104 (10.9822, 50.0761) -> (10.5729, 50.0761)
  arc A371 (10.5729, 50.0952) -> (10.5729, 50.0571) centre (10.5729, 50.0762) ccw
  arc A372 (16.491, 16.105) -> (16.4529, 16.105) centre (16.4719, 16.105) ccw
  line L105 (7.6073, 48.3574) -> (8.0984, 48.3574)
  line L106 (14.0589, 15.8186) -> (13.5678, 15.8186)
  line L107 (19.0119, 37.3592) -> (18.8482, 36.8681)
  arc A373 (8.1174, 48.6029) -> (8.0793, 48.6029) centre (8.0983, 48.6029) ccw
  arc A374 (7.8719, 48.0218) -> (7.8338, 48.0218) centre (7.8529, 48.0218) ccw
  line L108 (16.0627, 15.5321) -> (16.3082, 15.5321)
  arc A375 (15.7107, 16.2687) -> (15.6726, 16.2687) centre (15.6916, 16.2687) ccw
  arc A376 (7.9347, 48.0408) -> (7.9347, 48.0027) centre (7.9347, 48.0217) ccw
  arc A377 (11.3045, 50.0952) -> (11.3045, 50.0571) centre (11.3045, 50.0762) ccw
  arc A378 (12.3084, 50.6081) -> (12.2703, 50.6081) centre (12.2894, 50.6081) ccw
  arc A379 (7.8338, 47.6944) -> (7.8719, 47.6944) centre (7.8529, 47.6944) ccw
  arc A380 (10.7571, 50.7936) -> (10.7571, 50.8317) centre (10.7571, 50.8127) ccw
  arc A381 (7.9347, 48.0027) -> (7.9347, 48.0408) centre (7.9347, 48.0217) ccw
  line L109 (16.0627, 15.9413) -> (16.0627, 15.5321)
  arc A382 (7.7301, 47.6753) -> (7.7301, 47.7134) centre (7.7301, 47.6944) ccw
  arc A383 (7.9347, 47.6944) -> (7.9347, 48.0218) centre (7.9347, 47.8581) ccw
  arc A384 (7.6073, 47.8172) -> (7.7301, 47.6944) centre (7.7301, 47.8172) ccw
  arc A385 (12.4081, 16.0056) -> (12.3935, 16.0408) centre (12.4008, 16.0232) ccw
  arc A386 (12.7388, 15.8376) -> (12.7388, 15.7995) centre (12.7388, 15.8186) ccw
  arc A387 (11.9171, 15.8361) -> (11.9024, 15.801) centre (11.9097, 15.8186) ccw
  arc A388 (19.03, 37.3531) -> (18.9938, 37.3652) centre (19.0119, 37.3591) ccw
  line L110 (14.5021, 16.0641) -> (14.5021, 15.7367)
  arc A389 (7.9347, 47.7134) -> (7.9347, 47.6753) centre (7.9347, 47.6944) ccw
  arc A390 (14.9304, 16.2687) -> (14.8923, 16.2687) centre (14.9114, 16.2687) ccw
  arc A391 (16.1854, 15.9223) -> (16.1854, 15.9604) centre (16.1854, 15.9413) ccw
  arc A392 (14.9113, 16.2496) -> (14.9113, 16.2877) centre (14.9113, 16.2687) ccw
  arc A393 (8.0165, 48.622) -> (8.0165, 48.5839) centre (8.0165, 48.603) ccw
  line L111 (12.4008, 16.0232) -> (11.9097, 15.8186)
  arc A394 (12.2703, 50.117) -> (12.3084, 50.117) centre (12.2894, 50.117) ccw
  arc A395 (16.0627, 15.9604) -> (16.0627, 15.9223) centre (16.0627, 15.9413) ccw
  line L112 (12.5349, 50.3626) -> (12.0438, 50.3626)
  arc A396 (16.3082, 15.5321) -> (16.4719, 15.6958) centre (16.3082, 15.6958) ccw
  arc A397 (16.3082, 15.5512) -> (16.3082, 15.5131) centre (16.3082, 15.5321) ccw
  arc A398 (16.0627, 16.2877) -> (16.0627, 16.2496) centre (16.0627, 16.2687) ccw
  arc A399 (16.3082, 16.2496) -> (16.3082, 16.2877) centre (16.3082, 16.2687) ccw
  arc A400 (15.7083, 16.2594) -> (15.675, 16.278) centre (15.6917, 16.2687) ccw
  arc A401 (12.3935, 15.5964) -> (12.4081, 15.6315) centre (12.4008, 15.614) ccw
  line L113 (10.6343, 50.4853) -> (10.9822, 50.0761)
  line L114 (14.9113, 15.5321) -> (14.9113, 16.2687)
  arc A402 (7.6073, 48.3764) -> (7.6073, 48.3383) centre (7.6073, 48.3573) ccw
  arc A403 (18.8301, 36.8741) -> (18.8663, 36.8621) centre (18.8482, 36.8681) ccw
  arc A404 (10.592, 50.6286) -> (10.5539, 50.6285) centre (10.573, 50.6285) ccw
  line L115 (16.1854, 15.9413) -> (16.0627, 15.9413)
  line L116 (11.9097, 15.8186) -> (12.4008, 15.6139)
  arc A405 (11.0109, 43.6125) -> (11.0109, 43.6506) centre (11.0109, 43.6315) ccw
  arc A406 (10.301, 50.5611) -> (10.2648, 50.5732) centre (10.2829, 50.5671) ccw
  arc A407 (13.5678, 15.8376) -> (13.5678, 15.7995) centre (13.5678, 15.8186) ccw
  arc A408 (11.7137, 50.0571) -> (11.7137, 50.0952) centre (11.7137, 50.0762) ccw
  arc A409 (24.3177, 29.4527) -> (24.7269, 29.4527) centre (24.5223, 29.4527) ccw
  arc A410 (17.1265, 37.4001) -> (17.0884, 37.4001) centre (17.1075, 37.4001) ccw
  arc A411 (14.7067, 15.513) -> (14.7067, 15.5511) centre (14.7067, 15.5321) ccw
  arc A412 (17.8875, 37.6145) -> (17.8548, 37.5949) centre (17.8712, 37.6047) ccw
  arc A413 (17.1074, 37.0727) -> (17.5166, 37.0727) centre (17.312, 37.0727) ccw
  arc A414 (16.0817, 15.9413) -> (16.0436, 15.9413) centre (16.0627, 15.9413) ccw
  arc A415 (18.1004, 37.2053) -> (18.133, 37.1857) centre (18.1167, 37.1955) ccw
  arc A416 (17.4976, 37.4001) -> (17.5357, 37.4001) centre (17.5166, 37.4001) ccw
  line L117 (18.1167, 37.1955) -> (17.8712, 37.6047)
  line L118 (17.8712, 37.6047) -> (17.8712, 36.8681)
  arc A417 (16.4247, 37.6238) -> (16.4247, 37.5857) centre (16.4247, 37.6048) ccw
  line L119 (24.7269, 29.9847) -> (24.7269, 29.4527)
  arc A418 (16.6483, 37.6047) -> (16.6102, 37.6047) centre (16.6292, 37.6047) ccw
  arc A419 (16.491, 15.6958) -> (16.4529, 15.6958) centre (16.4719, 15.6958) ccw
  arc A420 (16.0436, 15.5321) -> (16.0817, 15.5321) centre (16.0627, 15.5321) ccw
  arc A421 (17.5357, 37.0727) -> (17.4976, 37.0727) centre (17.5166, 37.0727) ccw
  arc A422 (24.746, 29.4527) -> (24.7079, 29.4527) centre (24.727, 29.4527) ccw
  arc A423 (16.4529, 16.105) -> (16.491, 16.105) centre (16.4719, 16.105) ccw
  arc A424 (24.7079, 29.4527) -> (24.746, 29.4527) centre (24.727, 29.4527) ccw
  arc A425 (23.5028, 29.2541) -> (23.5389, 29.2421) centre (23.5208, 29.2481) ccw
  arc A426 (16.0627, 15.5512) -> (16.0627, 15.5131) centre (16.0627, 15.5321) ccw
  arc A427 (23.229, 29.9847) -> (23.1909, 29.9847) centre (23.21, 29.9847) ccw
  arc A428 (14.7067, 16.2877) -> (14.7067, 16.2496) centre (14.7067, 16.2687) ccw
  line L120 (23.21, 29.9847) -> (23.0054, 29.9847)
  arc A429 (18.3813, 37.6047) -> (18.3432, 37.6047) centre (18.3622, 37.6047) ccw
  arc A430 (14.7067, 16.2687) -> (14.5021, 16.0641) centre (14.7067, 16.0641) ccw
  line L121 (16.6293, 36.8681) -> (16.6293, 37.6047)
  arc A431 (17.0884, 37.0727) -> (17.1265, 37.0727) centre (17.1075, 37.0727) ccw
  arc A432 (18.7026, 37.3652) -> (18.6665, 37.3531) centre (18.6846, 37.3591) ccw
  arc A433 (15.2657, 15.5414) -> (15.299, 15.5228) centre (15.2824, 15.5321) ccw
  arc A434 (14.0589, 15.7995) -> (14.0589, 15.8376) centre (14.0589, 15.8186) ccw
  arc A435 (18.3786, 37.5949) -> (18.3459, 37.6145) centre (18.3623, 37.6047) ccw
  arc A436 (23.7845, 29.9907) -> (23.7483, 29.9787) centre (23.7664, 29.9847) ccw
  arc A437 (17.1265, 37.0727) -> (17.0884, 37.0727) centre (17.1075, 37.0727) ccw
  line L122 (23.7664, 29.9847) -> (23.5209, 29.2481)
  arc A438 (15.6726, 15.5321) -> (15.7107, 15.5321) centre (15.6916, 15.5321) ccw
  arc A439 (18.8301, 36.8621) -> (18.8663, 36.8741) centre (18.8482, 36.8681) ccw
  arc A440 (16.3082, 15.5131) -> (16.3082, 15.5512) centre (16.3082, 15.5321) ccw
  line L123 (15.6916, 15.5321) -> (15.6916, 16.2687)
  line L124 (14.7067, 15.5321) -> (14.9113, 15.5321)
  arc A441 (13.2298, 15.7995) -> (13.2298, 15.8376) centre (13.2298, 15.8186) ccw
  arc A442 (17.4976, 37.0727) -> (17.5357, 37.0727) centre (17.5166, 37.0727) ccw
  arc A443 (17.8521, 36.8681) -> (17.8902, 36.8681) centre (17.8712, 36.8681) ccw
  arc A444 (15.2633, 15.5321) -> (15.3014, 15.5321) centre (15.2824, 15.5321) ccw
  arc A445 (14.4831, 15.7367) -> (14.5212, 15.7367) centre (14.5022, 15.7367) ccw
  arc A446 (16.4719, 16.105) -> (16.3082, 16.2687) centre (16.3082, 16.105) ccw
  line L125 (17.1074, 37.4001) -> (17.1074, 37.0727)
  arc A447 (23.0054, 29.9657) -> (23.0054, 30.0038) centre (23.0054, 29.9847) ccw
  line L126 (13.2298, 15.8186) -> (12.7388, 15.8186)
  line L127 (18.3622, 37.6047) -> (18.1167, 37.1955)
  line L128 (16.3082, 16.2687) -> (16.0627, 16.2687)
  line L129 (15.6916, 16.2687) -> (15.2824, 15.5321)
  arc A448 (14.8923, 15.5321) -> (14.9304, 15.5321) centre (14.9114, 15.5321) ccw
  line L130 (22.8008, 29.2481) -> (22.9644, 29.5755)
  arc A449 (14.5212, 15.7367) -> (14.4831, 15.7367) centre (14.5022, 15.7367) ccw
  arc A450 (14.7067, 15.5512) -> (14.7067, 15.5131) centre (14.7067, 15.5321) ccw
  arc A451 (14.7067, 16.2496) -> (14.7067, 16.2877) centre (14.7067, 16.2687) ccw
  line L131 (14.9113, 16.2687) -> (14.7067, 16.2687)
  arc A452 (15.3014, 16.2687) -> (15.2633, 16.2687) centre (15.2824, 16.2687) ccw
  arc A453 (14.5021, 15.7367) -> (14.7067, 15.5321) centre (14.7067, 15.7367) ccw
  arc A454 (18.1004, 37.1857) -> (18.133, 37.2053) centre (18.1167, 37.1955) ccw
  arc A455 (16.8339, 37.5857) -> (16.8339, 37.6238) centre (16.8339, 37.6048) ccw
  arc A456 (14.5212, 16.0641) -> (14.4831, 16.0641) centre (14.5022, 16.0641) ccw
  line L132 (23.5822, 29.4322) -> (23.9505, 29.4322)
  arc A457 (22.9815, 29.567) -> (22.9474, 29.584) centre (22.9644, 29.5755) ccw
  arc A458 (21.971, 27.6483) -> (21.9274, 27.6221) centre (21.9492, 27.6352) ccw
  arc A459 (16.6102, 36.8681) -> (16.6483, 36.8681) centre (16.6292, 36.8681) ccw
  arc A460 (21.0582, 26.289) -> (21.0582, 26.3398) centre (21.0582, 26.3144) ccw
  line L133 (21.0582, 27.6352) -> (20.7647, 27.6352)
  arc A461 (21.3771, 26.6079) -> (21.3263, 26.6079) centre (21.3517, 26.6079) ccw
  arc A462 (24.0792, 27.6098) -> (24.0792, 27.6606) centre (24.0792, 27.6352) ccw
  arc A463 (21.0582, 27.6606) -> (21.0582, 27.6098) centre (21.0582, 27.6352) ccw
  arc A464 (23.6756, 25.4762) -> (23.6756, 25.527) centre (23.6756, 25.5016) ccw
  arc A465 (24.055, 25.2003) -> (24.1034, 25.2159) centre (24.0792, 25.2081) ccw
  arc A466 (23.3454, 27.6606) -> (23.3454, 27.6098) centre (23.3454, 27.6352) ccw
  arc A467 (21.3771, 27.3417) -> (21.3263, 27.3417) centre (21.3517, 27.3417) ccw
  arc A468 (23.3454, 25.1714) -> (23.4555, 24.9146) centre (23.7, 25.1714) ccw
  arc A469 (24.2986, 29.4527) -> (24.3367, 29.4527) centre (24.3177, 29.4527) ccw
  arc A470 (23.3708, 25.1714) -> (23.32, 25.1714) centre (23.3454, 25.1714) ccw
  arc A471 (23.0054, 29.5564) -> (23.0054, 29.5945) centre (23.0054, 29.5755) ccw
  arc A472 (23.6869, 26.3144) -> (23.7377, 26.3144) centre (23.7123, 26.3144) ccw
  arc A473 (23.9938, 29.2421) -> (24.03, 29.2541) centre (24.0119, 29.2481) ccw
  arc A474 (21.0582, 26.3398) -> (21.0582, 26.289) centre (21.0582, 26.3144) ccw
  arc A475 (23.6756, 25.5016) -> (23.3454, 25.1714) centre (23.6756, 25.1714) ccw
  arc A476 (23.32, 25.1714) -> (23.3708, 25.1714) centre (23.3454, 25.1714) ccw
  arc A477 (24.0792, 25.2081) -> (23.6756, 25.5016) centre (23.6756, 25.0774) ccw
  arc A478 (21.3263, 26.6079) -> (21.3771, 26.6079) centre (21.3517, 26.6079) ccw
  line L134 (18.3622, 36.8681) -> (18.3622, 37.6047)
  arc A479 (22.1231, 30.0038) -> (22.1231, 29.9657) centre (22.1231, 29.9847) ccw
  arc A480 (24.3367, 29.9847) -> (24.2986, 29.9847) centre (24.3177, 29.9847) ccw
  arc A481 (22.5323, 29.9657) -> (22.5323, 30.0038) centre (22.5323, 29.9847) ccw
  arc A482 (22.3087, 29.2481) -> (22.3468, 29.2481) centre (22.3278, 29.2481) ccw
  arc A483 (22.3468, 29.9847) -> (22.3087, 29.9847) centre (22.3278, 29.9847) ccw
  arc A484 (23.21, 29.9657) -> (23.21, 30.0038) centre (23.21, 29.9847) ccw
  line L135 (22.3277, 29.2481) -> (22.3277, 29.9847)
  arc A485 (21.3517, 27.3417) -> (21.0582, 27.6352) centre (21.0582, 27.3417) ccw
  arc A486 (22.8552, 27.6352) -> (22.8043, 27.6352) centre (22.8298, 27.6352) ccw
  arc A487 (22.8043, 26.3144) -> (22.8552, 26.3144) centre (22.8298, 26.3144) ccw
  arc A488 (23.6756, 25.527) -> (23.6756, 25.4762) centre (23.6756, 25.5016) ccw
  arc A489 (23.1909, 29.2481) -> (23.229, 29.2481) centre (23.21, 29.2481) ccw
  arc A490 (23.0054, 29.5945) -> (23.0054, 29.5564) centre (23.0054, 29.5755) ccw
  arc A491 (18.3432, 36.8681) -> (18.3813, 36.8681) centre (18.3622, 36.8681) ccw
  arc A492 (24.746, 29.9847) -> (24.7079, 29.9847) centre (24.727, 29.9847) ccw
  arc A493 (23.0054, 29.9847) -> (23.0054, 29.5755) centre (23.0054, 29.7801) ccw
  line L136 (23.0054, 29.5755) -> (23.21, 29.5755)
  arc A494 (22.7837, 29.2566) -> (22.8178, 29.2396) centre (22.8008, 29.2481) ccw
  line L137 (22.8298, 27.6352) -> (22.3895, 26.9014)
  arc A495 (23.7845, 29.9787) -> (23.7483, 29.9907) centre (23.7664, 29.9847) ccw
  arc A496 (17.8902, 37.6047) -> (17.8521, 37.6047) centre (17.8712, 37.6047) ccw
  arc A497 (24.3367, 29.4527) -> (24.2986, 29.4527) centre (24.3177, 29.4527) ccw
  line L138 (22.8298, 26.3144) -> (22.8298, 27.6352)
  arc A498 (21.3263, 27.3417) -> (21.3771, 27.3417) centre (21.3517, 27.3417) ccw
  line L139 (24.3177, 29.4527) -> (24.3177, 29.9847)
  arc A499 (23.21, 29.5564) -> (23.21, 29.5945) centre (23.21, 29.5755) ccw
  arc A500 (20.7647, 27.6606) -> (20.7647, 27.6098) centre (20.7647, 27.6352) ccw
  line L140 (24.0119, 29.2481) -> (23.7664, 29.9847)
  arc A501 (17.5357, 37.4001) -> (17.4976, 37.4001) centre (17.5166, 37.4001) ccw
  arc A502 (22.3677, 26.9145) -> (22.4113, 26.8884) centre (22.3895, 26.9015) ccw
  arc A503 (17.5166, 37.4001) -> (17.1074, 37.4001) centre (17.312, 37.4001) ccw
  arc A504 (23.5822, 29.4513) -> (23.5822, 29.4132) centre (23.5822, 29.4323) ccw
  arc A505 (17.0884, 37.4001) -> (17.1265, 37.4001) centre (17.1075, 37.4001) ccw
  line L141 (16.8339, 37.6047) -> (16.4247, 37.6047)
  line L142 (18.8482, 36.8681) -> (18.6845, 37.3592)
  arc A506 (23.9505, 29.4132) -> (23.9505, 29.4513) centre (23.9505, 29.4323) ccw
  line L143 (23.21, 29.2481) -> (23.21, 29.9847)
  arc A507 (23.0054, 30.0038) -> (23.0054, 29.9657) centre (23.0054, 29.9847) ccw
  line L144 (17.5166, 37.0727) -> (17.5166, 37.4001)
  line L145 (22.5323, 29.9847) -> (22.1231, 29.9847)
  arc A508 (21.4995, 24.1643) -> (21.5382, 24.1973) centre (21.5189, 24.1808) ccw
  arc A509 (21.0582, 27.6098) -> (21.0582, 27.6606) centre (21.0582, 27.6352) ccw
  arc A510 (20.7647, 26.3398) -> (20.7647, 26.289) centre (20.7647, 26.3144) ccw
  arc A511 (22.0653, 24.2062) -> (22.0653, 24.1554) centre (22.0653, 24.1808) ccw
  arc A512 (22.0399, 25.1714) -> (22.0907, 25.1714) centre (22.0653, 25.1714) ccw
  line L146 (22.799, 24.1808) -> (22.0653, 24.1808)
  line L147 (21.5189, 24.1808) -> (20.7851, 24.1808)
  arc A513 (19.7985, 24.8892) -> (19.7985, 24.94) centre (19.7985, 24.9146) ccw
  arc A514 (22.7749, 25.2003) -> (22.8232, 25.2159) centre (22.799, 25.2081) ccw
  line L148 (24.0792, 24.1808) -> (23.3454, 24.1808)
  arc A515 (20.8105, 25.1714) -> (20.7597, 25.1714) centre (20.7851, 25.1714) ccw
  arc A516 (20.9145, 24.931) -> (20.8758, 24.8981) centre (20.8952, 24.9146) ccw
  arc A517 (22.8515, 27.6221) -> (22.808, 27.6483) centre (22.8297, 27.6352) ccw
  arc A518 (21.1153, 25.4762) -> (21.1153, 25.527) centre (21.1153, 25.5016) ccw
  arc A519 (22.1947, 24.931) -> (22.156, 24.8981) centre (22.1753, 24.9146) ccw
  arc A520 (21.9746, 27.6352) -> (21.9238, 27.6352) centre (21.9492, 27.6352) ccw
  arc A521 (21.1153, 25.527) -> (21.1153, 25.4762) centre (21.1153, 25.5016) ccw
  arc A522 (20.2387, 25.4762) -> (20.2387, 25.527) centre (20.2387, 25.5016) ccw
  line L149 (23.7123, 26.3144) -> (23.7123, 27.6352)
  arc A523 (22.0653, 25.1714) -> (22.1753, 24.9146) centre (22.4198, 25.1713) ccw
  arc A524 (24.0792, 24.1554) -> (24.0792, 24.2062) centre (24.0792, 24.1808) ccw
  arc A525 (20.8777, 24.8962) -> (20.9127, 24.933) centre (20.8952, 24.9146) ccw
  arc A526 (19.505, 25.527) -> (19.505, 25.4762) centre (19.505, 25.5016) ccw
  arc A527 (22.3955, 25.4762) -> (22.3955, 25.527) centre (22.3955, 25.5016) ccw
  arc A528 (19.5304, 24.6211) -> (19.4796, 24.6211) centre (19.505, 24.6211) ccw
  arc A529 (22.7797, 24.1643) -> (22.8184, 24.1973) centre (22.7991, 24.1808) ccw
  arc A530 (19.7985, 24.1554) -> (19.7985, 24.2062) centre (19.7985, 24.1808) ccw
  line L150 (21.9492, 27.6352) -> (21.9492, 26.3144)
  arc A531 (19.5304, 24.4743) -> (19.4796, 24.4743) centre (19.505, 24.4743) ccw